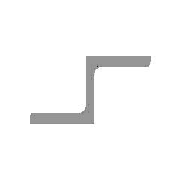
# Autodesk Inventor part: DIN1027 - Z 200 - 2040
Saved by Autodesk Inventor 2020 (Build 240168000, 168)
## iProperties
_CCFamilyMember: 11
_CCFamilyDisplayName: DIN 1027 Z - Zee-Shape
_FrameMemberDoc: Frame Member File
_Version: 15.0.0
_GetPNFromCC: 1
Created: 2018-08-31
Part Number: DIN1027 - Z 200 - 2040
Material: Steel, Mild
Description: Zee-Shape
Document SubType Name: Modeling
Standard: DIN
Designer: alid
Standard Revision: 2004
Standards Organization: DIN
Language: en-US
Size Designation: Z 200
Categories: <MemberInstance><Categories><Category DisplayName="Structural Shapes" InternalName="089c4875-fa83-4c05-b084-43b9cc11f5ed" Mnemonic="GRDR"><CategoryParameter DisplayName="Mass per Length Unit" InternalName="0bb95a10-148f-4027-a459-38d7b056702a" Mnemonic="shpmass"/><CategoryParameter DisplayName="Section Area" InternalName="1ff91680-64b0-4202-b9a3-7fd3f94bba3b" Mnemonic="secarea"/><CategoryParameter DisplayName="Radius of Gyration (x)" InternalName="25778675-03e9-40c1-b6a8-4a9ed693320d" Mnemonic="gyrradx"/><CategoryParameter DisplayName="Torsional Rigidity Modulus" InternalName="26c1ec35-5026-4c63-ad0a-751cf684a536" Mnemonic="torrigmod"/><CategoryParameter DisplayName="Distance of the Center of Gravity X-X" InternalName="26c9bdb8-9c79-4b4f-a92e-8e197583c9c4" Mnemonic="grcendistX"/><CategoryParameter DisplayName="Legacy Member ID" InternalName="340afe4f-75d7-48d3-ab7d-943f3c3da468" Mnemonic="LegacyMemberID"/><CategoryParameter DisplayName="Base Length" InternalName="42e34263-8f20-4d0e-ad48-bf1385b87c24" Mnemonic="shplen"/><CategoryParameter DisplayName="Moment of Inertia (y)" InternalName="4b9f58ea-bced-460e-81ea-3d29ca5a49e3" Mnemonic="inermomy"/><CategoryParameter DisplayName="Moment of Inertia (x)" InternalName="4cd780bc-73d7-43ac-917a-579e5cbd684d" Mnemonic="inermomx"/><CategoryParameter DisplayName="Custom Base Point" InternalName="4f1d1b73-316d-484b-a3df-9cbabb16eb77" Mnemonic="shpBasePoint"/><CategoryParameter DisplayName="Shape Height" InternalName="50274e7d-5ac0-4796-92cb-c59e54983c67" Mnemonic="shpheig"/><CategoryParameter DisplayName="Section Module (y)" InternalName="59eaa5e9-d227-48dc-b6c1-6920f96e0f95" Mnemonic="secmody"/><CategoryParameter DisplayName="Section Designation" InternalName="5a64d034-428d-49c8-ba32-7619764de20f" Mnemonic="shpdes"/><CategoryParameter DisplayName="Section Module (x)" InternalName="72cfad18-cf51-4ed4-aaa7-c6b224f8419f" Mnemonic="secmodx"/><CategoryParameter DisplayName="Torsional Section Modulus" InternalName="7c55a8dc-8844-49f9-a867-cc677b30ec9a" Mnemonic="torsecmod"/><CategoryParameter DisplayName="Shape Width" InternalName="7c717d54-a18f-4666-b4d4-573cce22c62c" Mnemonic="shpwdth"/><CategoryParameter DisplayName="Second Shape Thickness" InternalName="9251a8e1-85fd-4e47-af99-afdb762317d9" Mnemonic="shpthick2"/><CategoryParameter DisplayName="FG Authored" InternalName="9c666724-f362-4ea7-ac62-f6a007de5c69" Mnemonic="shpFGAuto"/><CategoryParameter DisplayName="Distance of the Center of Gravity Y-Y" InternalName="bcc4fb17-7af4-436a-8f8c-d0aa3b0248c5" Mnemonic="grcendistY"/><CategoryParameter DisplayName="Radius of Gyration (y)" InternalName="bfa18ebe-1636-4dbe-8d42-b263e0b73184" Mnemonic="gyrrady"/><CategoryParameter DisplayName="Shape Thickness" InternalName="d109cf76-8eb4-42fc-9800-4409734adc67" Mnemonic="shpthick"/><CategoryParameter DisplayName="Coefficient of Shear Displacement" InternalName="de4c90c6-aaa8-468f-a335-6737b311b5d3" Mnemonic="shdispc"/><Category DisplayName="Zees" InternalName="f2d48265-1196-4284-8641-bf60c20e8795" Mnemonic="ZSHP"><CategoryParameter DisplayName="Section Module (x)" InternalName="3836bdc1-0cd8-45f6-a1cd-1a678c824de9" Mnemonic="secmodx"/><CategoryParameter DisplayName="Radius of Gyration (y)" InternalName="3b80c782-6a7e-42a4-a61f-2934a0a3dd74" Mnemonic="gyrrady"/><CategoryParameter DisplayName="Moment of Inertia (x)" InternalName="48f5d714-e134-435c-9d71-5443f7fa7659" Mnemonic="inermomx"/><CategoryParameter DisplayName="Shape Width" InternalName="49a3dc8e-e4f5-40a7-a4e7-348596ff507c" Mnemonic="shpwdth"/><CategoryParameter DisplayName="Radius of Gyration (x)" InternalName="5257d526-50f9-4e95-b011-c72e627ab059" Mnemonic="gyrradx"/><CategoryParameter DisplayName="Section Area" InternalName="86aef8e9-359b-48d7-9b72-7721b6ddf74a" Mnemonic="secarea"/><CategoryParameter DisplayName="Section Module (y)" InternalName="890b9b56-5889-4192-8a12-a494904ebc04" Mnemonic="secmody"/><CategoryParameter DisplayName="Moment of Inertia (y)" InternalName="b68c6a0d-4456-4f11-b202-762159bb55c7" Mnemonic="inermomy"/><CategoryParameter DisplayName="Shape Thickness" InternalName="e1e0a9a7-d902-413f-ae78-d6cc14ea2e5c" Mnemonic="shpthick"/></Category></Category><Category DisplayName="DataType" InternalName="23b78d0f-2648-40c6-8793-ca6db495c9e8" Mnemonic="DATATYPE"><CategoryParameter DisplayName="DisplayName" InternalName="05415f3d-3907-474b-a020-eb9d644f4cf3" Mnemonic="DISPLAYNAME"/><CategoryParameter DisplayName="Standard" InternalName="0c0a119c-1e12-4c84-803f-101930972f5e" Mnemonic="STANDARD"/><CategoryParameter DisplayName="Description" InternalName="13903e3d-64b1-4950-80da-f627842ea37f" Mnemonic="DESCRIPTION"/><CategoryParameter DisplayName="Designation" InternalName="2675968c-4ce5-49e0-a4f5-552d29089031" Mnemonic="DESIGNATION"/><CategoryParameter DisplayName="Default Row" InternalName="2af9ec52-faaa-4026-b378-f9fa4afca842" Mnemonic="DEFAULTROW"/><CategoryParameter DisplayName="Folder Name" InternalName="3f06958e-8713-4116-9be7-ed6184ecc97b" Mnemonic="FOLDERNAME"/><CategoryParameter DisplayName="Revision Guid" InternalName="45a75005-10b1-4dfc-8d6d-dfe629f0b93c" Mnemonic="REVISIONGUID"/><CategoryParameter DisplayName="FileName" InternalName="8b46a4cc-9585-4fed-90c3-899f57e09a73" Mnemonic="FILENAME"/><CategoryParameter DisplayName="StdsOrg" InternalName="8f5914e1-4693-403f-8ab5-d37768198c9d" Mnemonic="STDSORG"/><CategoryParameter DisplayName="Family Version" InternalName="914462f6-6e19-4b14-ba84-155b9680b1d0" Mnemonic="FAMILYREVISION"/><CategoryParameter DisplayName="Standard Revision" InternalName="91d5a463-65c2-4fde-b823-3b7fea5e8e17" Mnemonic="STANDARDREVISION"/><CategoryParameter DisplayName="Member Revision" InternalName="a65d44b9-392f-4f4f-857b-e4b3d54996fe" Mnemonic="MEMBERREVISION"/><CategoryParameter DisplayName="ClipFormat" InternalName="bc51e27b-3422-4e78-93ef-cec197ddf230" Mnemonic="CLIPFORMAT"/><CategoryParameter DisplayName="Manufacturer" InternalName="cd6c7a72-a28a-4e50-99a9-2c7f4e13e5ad" Mnemonic="MANUFACTURER"/><CategoryParameter DisplayName="InternalName" InternalName="cf1d0246-76d9-4b4a-8305-fa0409afb5c1" Mnemonic="INTERNALNAME"/><CategoryParameter DisplayName="IsMetric" InternalName="e2385c5b-1ea4-4823-96a8-8de651266ec3" Mnemonic="ISMETRIC"/><Category DisplayName="Part" InternalName="c0e0b642-3bcb-4cc8-9e80-f96d35c4afa4" Mnemonic="PART"><CategoryParameter DisplayName="Part Number" InternalName="016b6077-bfbe-49bd-92c9-d8d59c39c941" Mnemonic="PARTNUMBER"/><CategoryParameter DisplayName="Stock Number" InternalName="4dba7c1c-e26c-444e-836c-b08b433409a8" Mnemonic="STOCKNUMBER"/><CategoryParameter DisplayName="Material Key" InternalName="5c9a8adb-dd2b-4535-b97f-0a94a95fe41f" Mnemonic="MATERIALKEY"/><CategoryParameter DisplayName="Material" InternalName="818a152a-d3c3-49ca-80ee-df7d91421b8e" Mnemonic="MATERIAL"/></Category></Category><Category DisplayName="LegacyMap" InternalName="cd87c42b-3e48-431e-b5c0-1cbeb14dfe77" Mnemonic="LEGACYMAP"><CategoryParameter DisplayName="unique DA member ID" InternalName="0918ad47-427f-4fed-ae26-24c81c58f590" Mnemonic="DACOOKIE"/><CategoryParameter DisplayName="Merge11 ID" InternalName="0ee8fb18-e2ed-4f39-96f6-1f4b5f50aa71" Mnemonic="MERGE11"/><CategoryParameter DisplayName="unique CC member ID" InternalName="5193edd4-b2b0-4ab4-9d54-de900eee34e0" Mnemonic="CCCOOKIE"/><CategoryParameter DisplayName="Split ID" InternalName="72b5c83c-be7f-45c4-ae51-9160ea6deb26" Mnemonic="SPLIT"/><CategoryParameter DisplayName="MemberID" InternalName="8e5e0294-fc51-4c8f-b3d7-003dc5ed94f6" Mnemonic="MEMBERID"/><CategoryParameter DisplayName="CatalogName" InternalName="d99d1e27-aa94-4de2-af4c-c348882a6f4f" Mnemonic="CATALOGNAME"/><CategoryParameter DisplayName="FamilyNumber" InternalName="e705e1f4-09cb-413e-91f9-551b4188271e" Mnemonic="FAMILYNUMBER"/></Category></Categories><FamilyTemplate Id="gp0501"><FamilyTemplateParameters><FamilyTemplateParameter ObjectType="kUserParameterObject" ValueType="xs:double" Id="1" ObjectReferenceKey="G_T1"/><FamilyTemplateParameter ObjectType="kUserParameterObject" ValueType="xs:double" Id="3" ObjectReferenceKey="G_ER"/><FamilyTemplateParameter ObjectType="kUserParameterObject" ValueType="xs:double" Id="4" ObjectReferenceKey="G_H"/><FamilyTemplateParameter ObjectType="kUserParameterObject" ValueType="xs:double" Id="5" ObjectReferenceKey="B_L"/><FamilyTemplateParameter ObjectType="kUserParameterObject" ValueType="xs:double" Id="8" ObjectReferenceKey="G_W"/><FamilyTemplateParameter ObjectType="kUserParameterObject" ValueType="xs:double" Id="9" ObjectReferenceKey="G_T"/><FamilyTemplateParameter ObjectType="kUserParameterObject" ValueType="xs:double" Id="10" ObjectReferenceKey="G_IR"/><FamilyTemplateParameter ObjectType="kPropertyObject" ValueType="xs:string" Id="100" ObjectReferenceKey="{32853F0F-3444-11d1-9E93-0060B03C1CA6}" SubObjectId="52"/><FamilyTemplateParameter ObjectType="kPropertyObject" ValueType="xs:string" Id="105" ObjectReferenceKey="{32853F0F-3444-11d1-9E93-0060B03C1CA6}" SubObjectId="5"/><FamilyTemplateParameter ObjectType="kPartComponentDefinitionObject" ValueType="xs:string" Id="110" SubObjectId="Material"/><FamilyTemplateParameter ObjectType="kPropertyObject" ValueType="xs:string" Id="112" ObjectReferenceKey="{32853F0F-3444-11d1-9E93-0060B03C1CA6}" SubObjectId="55"/></FamilyTemplateParameters></FamilyTemplate><CategoryParameterMap><ParamToTemplateMap><ParamToTemplate CategoryParameter="//CategoryParameter[@InternalName='05415f3d-3907-474b-a020-eb9d644f4cf3']" ConstantValue="DIN 1027 Z"/><ParamToTemplate CategoryParameter="//CategoryParameter[@InternalName='cf1d0246-76d9-4b4a-8305-fa0409afb5c1']" ConstantValue="20ab7e12-1fb4-424f-b041-298e7a290ef0"/><ParamToTemplate CategoryParameter="//CategoryParameter[@InternalName='3f06958e-8713-4116-9be7-ed6184ecc97b']" ConstantValue="DIN 1027  Z"/><ParamToTemplate CategoryParameter="//CategoryParameter[@InternalName='914462f6-6e19-4b14-ba84-155b9680b1d0']" ConstantValue="10"/><ParamToTemplate CategoryParameter="//CategoryParameter[@InternalName='bc51e27b-3422-4e78-93ef-cec197ddf230']" ConstantValue="CF_INVENTOR.STDPARTS"/><ParamToTemplate CategoryParameter="//CategoryParameter[@InternalName='e2385c5b-1ea4-4823-96a8-8de651266ec3']" ConstantValue="true"/><ParamToTemplate CategoryParameter="//CategoryParameter[@InternalName='13903e3d-64b1-4950-80da-f627842ea37f']" ConstantValue="Zee-Shape"/><ParamToTemplate CategoryParameter="//CategoryParameter[@InternalName='8f5914e1-4693-403f-8ab5-d37768198c9d']" ConstantValue="DIN"/><ParamToTemplate CategoryParameter="//CategoryParameter[@InternalName='0c0a119c-1e12-4c84-803f-101930972f5e']" ConstantValue="DIN 1027"/><ParamToTemplate CategoryParameter="//CategoryParameter[@InternalName='cd6c7a72-a28a-4e50-99a9-2c7f4e13e5ad']" TemplateParameter="104"/><ParamToTemplate CategoryParameter="//CategoryParameter[@InternalName='91d5a463-65c2-4fde-b823-3b7fea5e8e17']" ConstantValue="2004"/><ParamToTemplate CategoryParameter="//CategoryParameter[@InternalName='45a75005-10b1-4dfc-8d6d-dfe629f0b93c']" ConstantValue="cd1cf5ec-be03-4189-9927-10a4e7275960"/><ParamToTemplate CategoryParameter="//CategoryParameter[@InternalName='2af9ec52-faaa-4026-b378-f9fa4afca842']" ConstantValue="1"/><ParamToTemplate CategoryParameter="//CategoryParameter[@InternalName='9c666724-f362-4ea7-ac62-f6a007de5c69']" ConstantValue="1"/><ParamToTemplate CategoryParameter="//CategoryParameter[@InternalName='d99d1e27-aa94-4de2-af4c-c348882a6f4f']" ConstantValue="DIN"/><ParamToTemplate CategoryParameter="//CategoryParameter[@InternalName='e705e1f4-09cb-413e-91f9-551b4188271e']" ConstantValue="321"/><ParamToTemplate CategoryParameter="//CategoryParameter[@InternalName='8b46a4cc-9585-4fed-90c3-899f57e09a73']" ConstantValue="DIN1027 - Z 200 - 0.001"/><ParamToTemplate CategoryParameter="//CategoryParameter[@InternalName='a65d44b9-392f-4f4f-857b-e4b3d54996fe']" ConstantValue="1C69AECA-E285-4553-8F21-F3988829C810"/><ParamToTemplate CategoryParameter="//CategoryParameter[@InternalName='48f5d714-e134-435c-9d71-5443f7fa7659']" ConstantValue="2300"/><ParamToTemplate CategoryParameter="//CategoryParameter[@InternalName='5257d526-50f9-4e95-b011-c72e627ab059']" ConstantValue="7.71"/><ParamToTemplate CategoryParameter="//CategoryParameter[@InternalName='3b80c782-6a7e-42a4-a61f-2934a0a3dd74']" ConstantValue="3.04"/><ParamToTemplate CategoryParameter="//CategoryParameter[@InternalName='b68c6a0d-4456-4f11-b202-762159bb55c7']" ConstantValue="357"/><ParamToTemplate CategoryParameter="//CategoryParameter[@InternalName='3836bdc1-0cd8-45f6-a1cd-1a678c824de9']" ConstantValue="230"/><ParamToTemplate CategoryParameter="//CategoryParameter[@InternalName='890b9b56-5889-4192-8a12-a494904ebc04']" ConstantValue="47.6"/><ParamToTemplate CategoryParameter="//CategoryParameter[@InternalName='86aef8e9-359b-48d7-9b72-7721b6ddf74a']" ConstantValue="38.7"/><ParamToTemplate CategoryParameter="//CategoryParameter[@InternalName='5a64d034-428d-49c8-ba32-7619764de20f']" ConstantValue="Z 200"/><ParamToTemplate CategoryParameter="//CategoryParameter[@InternalName='8e5e0294-fc51-4c8f-b3d7-003dc5ed94f6']" ConstantValue="11"/><ParamToTemplate CategoryParameter="//CategoryParameter[@InternalName='42e34263-8f20-4d0e-ad48-bf1385b87c24']" TemplateParameter="5"/><ParamToTemplate CategoryParameter="//CategoryParameter[@InternalName='2675968c-4ce5-49e0-a4f5-552d29089031']" TemplateParameter="100"/><ParamToTemplate CategoryParameter="//CategoryParameter[@InternalName='50274e7d-5ac0-4796-92cb-c59e54983c67']" TemplateParameter="4"/><ParamToTemplate CategoryParameter="//CategoryParameter[@InternalName='818a152a-d3c3-49ca-80ee-df7d91421b8e']" TemplateParameter="110"/><ParamToTemplate CategoryParameter="//CategoryParameter[@InternalName='016b6077-bfbe-49bd-92c9-d8d59c39c941']" TemplateParameter="105"/><ParamToTemplate CategoryParameter="//CategoryParameter[@InternalName='4dba7c1c-e26c-444e-836c-b08b433409a8']" TemplateParameter="112"/></ParamToTemplateMap></CategoryParameterMap></MemberInstance>
Stock Number: Z 200
Density: 7.85 g/cm^3
Appearance: Semi-Polished
Mass: 101583 g
Surface Area: 22898.4 cm^2
Volume: 12940.5 cm^3
G_L: 2040.000 mm
G_W: 150.000 mm
G_H: 200.000 mm
+EC43E36D-5CDA-4CC5-8EE3-48E6D1311DAD+CUTDETAIL1: Cut Angle 90.00 deg
+2AA682CF-A4D9-41DF-907B-9091534C8CDF+CUTDETAIL2: Cut Angle 90.00 deg
IsCustomPart: 1
Author: alid
Autodesk Inventor part; units mm, degrees
ref_plane "YZ Plane" through (0, 0, 0) normal (1, 0, 0) x (0, 1, 0)
ref_plane "XZ Plane" through (0, 0, 0) normal (0, 1, 0) x (-1, 0, 0)
ref_plane "XY Plane" through (0, 0, 0) normal (0, 0, 1) x (1, 0, 0)
ref_plane "Start plane" through (0, 0, 80) normal (0, 0, 1) x (1, 0, 0)
ref_plane "End plane" through (0, 0, 2120) normal (0, 0, 1) x (1, 0, 0)
sketch "Sketch" plane through (0, 0, 0) normal (0, 0, 1) x (1, 0, 0)
  line L0 (-75, -100) -> (5, -100)
  line L1 (5, -100) -> (5, 74)
  line L2 (18, 87) -> (68.5, 87)
  line L3 (75, 93.5) -> (75, 100)
  line L4 (75, 100) -> (-5, 100)
  line L5 (-5, 100) -> (-5, -74)
  line L6 (-18, -87) -> (-68.5, -87)
  line L7 (-75, -93.5) -> (-75, -100)
  line L8 (173.6154, 0) -> (-40.1539, 0) construction
  line L9 (0, -212) -> (0, 68) construction
  arc A0 (-18, -87) -> (-5, -74) centre (-18, -74) ccw
  arc A1 (18, 87) -> (5, 74) centre (18, 74) ccw
  arc A2 (-68.5, -87) -> (-75, -93.5) centre (-68.5, -93.5) ccw
  arc A3 (68.5, 87) -> (75, 93.5) centre (68.5, 93.5) ccw
  line L10 (0, 162.4) -> (0, -274.4) construction
  line L11 (-126.3385, 0) -> (223.6078, 0) construction
  point P0 (5, 87)
  point P1 (75, 87)
  point P2 (-5, -87)
  point P3 (-75, -87)
  dimension "d0" = 200
  dimension "d1" = 80
  dimension "d2" = 80
  dimension "d3" = 13
  dimension "d4" = 13
  dimension "d5" = 10
  dimension "d10" = 13
  dimension "d11" = 6.5
  dimension "d12" = 5
  dimension "d13" = 100
  constraints: 20 end point, 8 point on circle, 8 point on line, 8 tangent, 6 parallel, 4 centre point, 2 collinear, 2 equal radius, 1 perpendicular
  measures "d0" distance between parallel lines of L0 L4
  measures "d1" distance between parallel lines of L5 L3
  measures "d2" distance between parallel lines of L7 L1
  measures "d3" distance between parallel lines of L0 L6
  measures "d4" distance between parallel lines of L2 L4
  measures "d5" distance between parallel lines of L5 L1
  measures "d10" radius of A0
  measures "d11" radius of A2
  measures "d12" distance between parallel lines of L5 L9
  measures "d13" distance between parallel lines of L4 L8
extrude "Body" add sketch "Sketch" along normal up to surface (2040 mm away) from surface at 80
sketch "Sketch3" plane through (0, 0, 0) normal (0, 0, 1) x (1, 0, 0)
  line L0 (0, 0) -> (10, 0)
ref_plane "Work Plane3" through (0, 0, 0) normal (0, -1, 0) x (1, 0, 0)
sketch "Sketch4" plane through (0, 0, 0) normal (0, -1, 0) x (1, 0, 0)
  line L0 (-2, 80) -> (12, 80)
  line L1 (-2, 2120) -> (12, 2120)
  dimension "d17" = 2040
  measures "d17" distance between parallel lines of L0 L1
ref_plane "Work Plane4" through (-1500, 0, 80) normal (0, 0, -1) x (-1, 0, 0)
split "Split1" plane through (-1500, 0, 80) removes the side toward (0, 0, -1)
ref_plane "Work Plane5" through (3500, 0, 2120) normal (0, 0, 1) x (1, 0, 0)
split "Split2" plane through (3500, 0, 2120) removes the side toward (0, 0, 1)
equation "\"d0\" = G_H"
equation "\"d1\" = G_W"
equation "\"d2\" = G_W"
equation "\"d3\" = G_T1"
equation "\"d4\" = G_T1"
equation "\"d5\" = G_T"
equation "\"d10\" = G_IR"
equation "\"d11\" = G_ER"
equation "\"d12\" = 0.5 * d5"
equation "\"d13\" = 0.5 * d0"
equation "\"d6\" = G_L"
equation "\"G_W\" = 80"
equation "\"G_H\" = 200"
equation "\"G_T\" = 10"
equation "\"G_T1\" = 13"
equation "\"G_IR\" = 13"
equation "\"G_ER\" = 6.5"
equation "\"G_L\" = d17"
body "Solid1"
